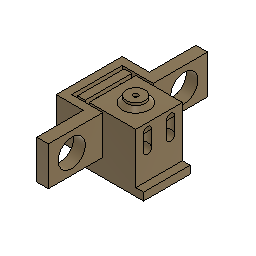
Heatblock+Mk2 (Autodesk Fusion 360 design; units mm, degrees)
Autodesk Fusion 360 part; units mm, degrees
sketch "Sketch1" plane through (0, 0, 0) normal (0, 0, 1) x (1, 0, 0)
  circle A0 centre (0, 0) radius 0.95
  line L0 (-6, 6) -> (6, 6)
  line L1 (6, 6) -> (6, -6)
  line L2 (6, -6) -> (-6, -6)
  line L3 (-6, -6) -> (-6, 6)
  line L4 (-6, 6) -> (6, -6) construction
  line L5 (6, 6) -> (-6, -6) construction
  dimension "d1" = 1.9
  dimension "d2" = 12
  dimension "d3" = 12
  constraint coincident A0.centre origin
  constraint horizontal L0
  constraint perpendicular L0 L1
  constraint parallel L0 L2
  constraint parallel L1 L3
  constraint coincident L4 A0.centre
  constraint coincident L5 A0.centre
  measures "d1" diameter of A0
  measures "d2" distance of L0.end L1.end
  measures "d3" distance of L1.end L2.end
extrude "Extrude1" add sketch "Sketch1" along normal blind 15 makes body 1
ref_plane "WorkPlane1" through (0, 0, 7.5) normal (-1, 0, 0) x (0, -1, 0)
sketch "Sketch2" plane through (0, 1.5, 5) normal (-1, 0, 0) x (0, 1, 0)
  line L0 (-0.55, -10) -> (-2.45, -10)
  line L1 (-7.5, -10) -> (4.5, -10)
  line L2 (4.5, -10) -> (-7.5, -10)
  line L3 (-1.5, -10) -> (-1.5, -12.3) construction
  line L4 (-1.5, -11) -> (-2.1, -11)
  line L5 (-1.5, -11) -> (-0.9, -11)
  line L6 (-0.9, -11) -> (-0.55, -10)
  line L7 (-2.1, -11) -> (-2.45, -10)
  line L8 (-4.9, -10) -> (-3.9, -11)
  line L9 (-3.9, -11) -> (-2.1, -11)
  line L10 (0.9, -11) -> (-0.9, -11)
  line L11 (1.9, -10) -> (0.9, -11)
  line L12 (-0.55, -10) -> (-2.45, -10)
  dimension "d7" = 0.6
  dimension "d23" = 1
  dimension "d24" = 45
  dimension "d25" = 1.8
  constraint midpoint L0 L3.start
  constraint perpendicular L1 L3
  constraint coincident L3 L4.start
  constraint perpendicular L3 L4
  constraint symmetric L3 L4.start L5.start
  constraint symmetric L3 L4.end L5.end
  constraint coincident L0.start L6.end
  constraint coincident L1 L8.start
  constraint parallel L4 L9
  constraint symmetric L3 L8.start L11.start
  constraint symmetric L3 L8.end L10.start
  constraint coincident L0.end L7
  measures "d7" distance of L4.start L4.end
  measures "d23" distance of L1 L9
  measures "d24" angle of L1 L8
  measures "d25" distance of L4.end L8.end
revolve "Revolve1" add sketch "Sketch2" angle 360 about axis through (0, 0, 15) along (0, 0, 1) contours L1 L2 L7 L8 L9 bodies 1
extrude "Extrude2" add 1 faces at (0.149, -1.7888, 16) along direction (0, 0, 1) blind 0.6 on bodies 1 bodies 1
sketch "Sketch3" plane through (6, 0, 0) normal (1, 0, 0) x (0, 1, 0)
  line L0 (-6, 0) -> (6, 0)
  line L1 (6, 15) -> (-6, 15)
  line L2 (-6, 15) -> (-6, 0)
  circle A0 centre (2.95, 13) radius 1.1
  line L3 (-0.95, 0) -> (0.95, 0)
  line L4 (0.95, 15) -> (6, 15)
  line L5 (0.95, 15) -> (0.95, 3) construction
  line L6 (2.95, 13) -> (0.95, 13) construction
  line L7 (2.95, 13) -> (2.95, 15) construction
  line L8 (-0.95, 15) -> (0.95, 15)
  line L9 (6, 0) -> (6, 15)
  line L10 (2.95, 13) -> (2.95, 9) construction
  circle A1 centre (2.95, 9) radius 1.1
  line L11 (0, 15) -> (0, 3.7377) construction
  line L12 (2.95, 9) -> (0.95, 9) construction
  circle A2 centre (-2.95, 13) radius 1.1
  circle A3 centre (-2.95, 9) radius 1.1
  dimension "d11" = 2.2
  dimension "d12" = 2
  dimension "d13" = 2
  dimension "d26" = 2.2
  dimension "d28" = 4
  constraint coincident L1.start L4.end
  constraint perpendicular L4 L5
  constraint coincident A0.centre L6.start
  constraint coincident L5 L6.end
  constraint perpendicular L5 L6
  constraint coincident L1 L7.end
  constraint perpendicular L1 L7
  constraint perpendicular L6 L10
  constraint coincident L10.end A1.centre
  constraint midpoint L8 L11.start
  constraint perpendicular L8 L11
  constraint midpoint L5 L12.end
  constraint horizontal L12
  constraint coincident L4.start L5
  constraint coincident L4.start L5.start
  constraint vertical L5
  constraint symmetric A0 L11 A2
  constraint symmetric A1 L11 A3
  measures "d11" diameter of A0
  measures "d12" distance of A0.centre L7.end
  measures "d13" distance of A0.centre L6.end
  measures "d26" diameter of A1
  measures "d28" distance of A0.centre L10.end
extrude "Extrude3" cut sketch "Sketch3" against normal blind 13.5 contours A0 | A1 | A2 | A3 bodies 1
sketch "Sketch7" plane through (0, -6, 0) normal (0, -1, 0) x (1, 0, 0)
  line L0 (-6, 0) -> (6, 0)
  line L1 (6, 0) -> (6, 15)
  line L2 (6, 15) -> (-6, 15)
  line L3 (-6, 15) -> (-6, 0)
  line L4 (6, 0) -> (8, 0)
  line L5 (8, 0) -> (8, 2)
  line L6 (8, 2) -> (6, 2)
  line L7 (6, 2) -> (6, 0)
  line L8 (-6, 0) -> (-8, 0)
  line L9 (-8, 0) -> (-8, 2)
  line L10 (-8, 2) -> (-6, 2)
  line L11 (-6, 2) -> (-6, 0)
  dimension "d17" = 2
  dimension "d18" = 2
  dimension "d19" = 2
  dimension "d20" = 2
  constraint horizontal L4
  constraint vertical L5
  constraint horizontal L6
  constraint vertical L7
  constraint coincident L0.end L1.start
  constraint horizontal L8
  constraint vertical L9
  constraint horizontal L10
  constraint vertical L11
  constraint coincident L0.start L3.end
  measures "d17" distance of L0.end L4.end
  measures "d18" distance of L0.end L6.end
  measures "d19" distance of L0.start L8.end
  measures "d20" distance of L0.start L10.end
extrude "Extrude4" add sketch "Sketch7" against normal blind 12 contours L3 L8 L9 L10 L11 | L1 L4 L5 L6 L7 bodies 1
sketch "Sketch9" plane through (0, 0, 15) normal (0, 0, 1) x (-1, 0, 0)
  circle A0 centre (0, 0) radius 3.4
  line L0 (6, 6) -> (-6, 6)
  line L1 (-6, 6) -> (-6, -6)
  line L2 (-6, -6) -> (6, -6)
  line L3 (6, -6) -> (6, 6)
  line L4 (-6, 1.85) -> (-6, 4.05)
  line L5 (-6, 6) -> (-6, -6)
  line L6 (-6, -6) -> (-6, 6)
  line L7 (-6, -4.05) -> (-6, -1.85)
  line L8 (-6, 1.85) -> (-6, 4.05)
  line L9 (-6, -4.05) -> (-6, -1.85)
  line L10 (-6, 1.85) -> (-6, 4.05)
  circle A1 centre (-6, 2.95) radius 1.1
  line L11 (-6, 0) -> (-8.5, 0)
  circle A2 centre (-6, -2.95) radius 1.1
  constraint midpoint L4 A1.centre
  constraint coincident L4.start A1
  constraint midpoint L6 L11.start
  constraint perpendicular L6 L11
  constraint symmetric A1 L11 A2
extrude "Extrude5" add sketch "Sketch9" along normal blind -6 and the other way blind 2 separate body contours L1 L4 L5 L6 L8 L10 A1 | L1 L4 L5 L6 L8 L10 A1 | L1 L5 L6 L7 L9 A2 | L1 L5 L6 L7 L9 A2 makes body 2 at (4.9055, -2.8405, 10.3333) makes body 3 at (4.9055, 3.0595, 10.3333)
ref_plane "WorkPlane3" through (0, 0, 7.5) normal (1, 0, 0) x (0, 1, 0)
mirror "Mirror1" about plane through (0, 0, 7.5) normal (1, 0, 0) of bodies 3 2 makes body 4 at (-4.9055, -2.8405, 10.3333) makes body 5 at (-4.9055, 3.0595, 10.3333)
combine "Combine1" operation cut target body 1 tool bodies 4 5 2 3
sketch "Sketch10" plane through (0, 6, 0) normal (0, 1, 0) x (-1, 0, 0)
  line L0 (-8, 0) -> (8, 0)
  line L1 (6, 2) -> (6, 15)
  line L2 (6, 15) -> (-6, 15)
  line L3 (-6, 15) -> (-6, 2)
  line L4 (-6, 15) -> (-7, 15)
  line L5 (-7, 15) -> (-7, 6)
  line L6 (-7, 6) -> (-6, 6)
  line L7 (-6, 6) -> (-6, 15)
  line L8 (-7, 15) -> (-9, 15)
  line L9 (-9, 15) -> (-9, 6)
  line L10 (-9, 6) -> (-7, 6)
  line L11 (-7, 6) -> (-7, 15)
  line L12 (0, 15) -> (0, 11.668)
  line L13 (9, 15) -> (9, 6)
  line L14 (9, 6) -> (7, 6)
  line L15 (7, 6) -> (7, 15)
  line L16 (7, 15) -> (9, 15)
  line L17 (8, 0) -> (8, 2)
  line L18 (8, 2) -> (6, 2)
  line L19 (-6, 2) -> (-8, 2)
  line L20 (-8, 2) -> (-8, 0)
  dimension "d35" = 1
  dimension "d36" = 9
  dimension "d37" = 2
  constraint horizontal L4
  constraint vertical L5
  constraint horizontal L6
  constraint vertical L7
  constraint coincident L2.end L3.start
  constraint horizontal L8
  constraint vertical L9
  constraint horizontal L10
  constraint vertical L11
  constraint midpoint L2 L12.start
  constraint perpendicular L2 L12
  constraint symmetric L4.end L12 L15.end
  constraint symmetric L8.end L12 L13.start
  constraint symmetric L9.end L12 L13.end
  constraint symmetric L5.end L12 L14.end
  measures "d35" distance of L2.end L4.end
  measures "d36" distance of L2.end L6.end
  measures "d37" distance of L4.end L8.end
extrude "Extrude6" add sketch "Sketch10" against normal blind 12 separate body contours L5 L8 L9 L10 L11 makes body 6
sketch "Sketch11" plane through (7, 0, 0) normal (-1, 0, 0) x (0, -1, 0)
  line L0 (-6, 15) -> (-6, 6)
  line L1 (-6, 6) -> (6, 6)
  line L2 (6, 6) -> (6, 15)
  line L3 (6, 15) -> (-6, 15)
  line L4 (-1.85, 13) -> (-1.85, 9)
  arc A0 (-4.05, 9) -> (-1.85, 9) centre (-2.95, 9) ccw
  line L5 (-4.05, 9) -> (-4.05, 13)
  arc A1 (-1.85, 13) -> (-4.05, 13) centre (-2.95, 13) ccw
  line L6 (4.05, 13) -> (4.05, 9)
  arc A2 (1.85, 9) -> (4.05, 9) centre (2.95, 9) ccw
  line L7 (1.85, 9) -> (1.85, 13)
  arc A3 (4.05, 13) -> (1.85, 13) centre (2.95, 13) ccw
  line L8 (-6, 2) -> (6, 2)
  line L9 (6, 2) -> (6, 15)
  line L10 (6, 15) -> (-6, 15)
  line L11 (-6, 15) -> (-6, 2)
  line L12 (-2.95, 13) -> (-2.95, 9) construction
  line L13 (-2.95, 11) -> (2.95, 11) construction
  line L14 (2.95, 13) -> (2.95, 9) construction
  line L15 (-2.95, 10) -> (2.95, 10)
  arc A4 (2.95, 10) -> (2.95, 12) centre (2.95, 11) ccw
  line L16 (2.95, 12) -> (-2.95, 12)
  arc A5 (-2.95, 12) -> (-2.95, 10) centre (-2.95, 11) ccw
  line L17 (-2.95, 11) -> (2.95, 11) construction
  line L18 (-1, 11) -> (-1, 6)
  arc A6 (-1, 6) -> (1, 6) centre (0, 6) ccw
  line L19 (1, 6) -> (1, 11)
  arc A7 (1, 11) -> (-1, 11) centre (0, 11) ccw
  line L20 (0, 11) -> (0, 6) construction
  dimension "d40" = 2
  dimension "d44" = 2
  constraint coincident A1.centre L12.start
  constraint coincident A0.centre L12.end
  constraint midpoint L12 L13.start
  constraint perpendicular L7 L13
  constraint coincident A3.centre L14.start
  constraint coincident A2.centre L14.end
  constraint coincident L13.end L14
  constraint tangent L15 A4
  constraint tangent A4 L16
  constraint parallel L15 L16
  constraint tangent L16 A5
  constraint tangent L15 A5
  constraint coincident L13.end A4.centre
  constraint perpendicular L14 L17
  constraint coincident L13.start A5.centre
  constraint tangent L18 A6
  constraint tangent A6 L19
  constraint parallel L18 L19
  constraint tangent L19 A7
  constraint tangent L18 A7
  constraint perpendicular L15 L20
  constraint midpoint L13 A7.centre
  measures "d40" diameter of A4
  measures "d44" diameter of A6
extrude "Extrude7" cut sketch "Sketch11" against normal blind 1 contours L1 L15 L18 L19 | L15 L18 L19 A7 | L4 L15 L16 L18 A7 | L7 L15 L16 L19 A7 | L4 L15 L16 A5 | L4 A0 L5 A1 L15 L16 A5 | L6 A2 L7 A3 L15 A4 L16 | L7 L15 A4 L16 bodies 6
sketch "Sketch12" plane through (0, 0, 6) normal (0, 0, -1) x (1, 0, 0)
  line L0 (7, 1) -> (8, 1)
  line L1 (8, 1) -> (8, -1)
  line L2 (8, -1) -> (7, -1)
  line L3 (7, -1) -> (7, -6)
  line L4 (7, -6) -> (9, -6)
  line L5 (9, -6) -> (9, 6)
  line L6 (9, 6) -> (7, 6)
  line L7 (7, 6) -> (7, 1)
  line L8 (8, 1) -> (9, 1)
  line L9 (9, 1) -> (9, -1)
  line L10 (9, -1) -> (8, -1)
  line L11 (8, -1) -> (8, 1)
  constraint horizontal L8
  constraint vertical L9
  constraint horizontal L10
  constraint vertical L11
  constraint coincident L5 L9.end
  constraint coincident L0.end L1.start
extrude "Extrude8" cut sketch "Sketch12" against normal blind 1 contours L1 L5 L8 L9 L10 L11 bodies 6
mirror "Mirror2" about plane through (0, 0, 0) normal (1, 0, 0) of bodies 6 makes body 7
move_face "OffsetFaces1" offset -0.3 1 faces at (0, -0.95, 5) on bodies 1
sketch "Sketch13" plane through (0, 0, 15) normal (0, 0, 1) x (-1, 0, 0)
  line L0 (-9, -6) -> (-7, -6)
  line L1 (-7, -6) -> (-7, 6)
  line L2 (-7, 6) -> (-9, 6)
  line L3 (-9, 6) -> (-9, -6)
  circle A0 centre (0, 0) radius 3.4
  line L4 (6, 6) -> (-6, 6)
  line L5 (-6, 6) -> (-6, -6)
  line L6 (-6, -6) -> (6, -6)
  line L7 (6, -6) -> (6, 6)
  line L8 (7, -6) -> (9, -6)
  line L9 (9, -6) -> (9, 6)
  line L10 (9, 6) -> (7, 6)
  line L11 (7, 6) -> (7, -6)
  line L12 (-10, 0.0008) -> (-10, -6.5)
  line L13 (-10, -6.5) -> (0, -6.5)
  line L14 (-11.9999, 0.0008) -> (-11.9999, -8.5001)
  line L15 (-11.9999, -8.5001) -> (-4.9999, -8.5001)
  line L16 (0, -6.5) -> (0, -6)
  line L17 (-11.9999, 0.0008) -> (-13.5981, 0.0008)
  line L18 (-2, -6.5) -> (-5, -6.5)
  line L19 (-4.9999, -8.5001) -> (-5, -8.5001)
  line L20 (-2, -8.4981) -> (-2, -6.5)
  line L21 (-5, -8.5001) -> (-5, -20.4981)
  line L22 (-5, -20.4981) -> (-2, -20.4981)
  line L23 (-2, -20.4981) -> (-2, -8.4981)
  line L24 (-11.9999, 0.0008) -> (-10, 0.0008)
  line L25 (-11.9999, 0.0008) -> (-11.9999, 8.5016)
  line L26 (-4.9999, 8.5016) -> (-5, 8.5016)
  line L27 (-5, 8.5016) -> (-5, 20.4996)
  line L28 (-5, 20.4996) -> (-2, 20.4996)
  line L29 (-2, 20.4996) -> (-2, 8.4996)
  line L30 (-2, 8.4996) -> (-2, 6.5015)
  line L31 (-11.9999, 8.5016) -> (-4.9999, 8.5016)
  line L32 (-11.9999, 0.0008) -> (-10, 0.0008)
  line L33 (-10, 0.0008) -> (-10, 6.5015)
  line L34 (-10, 6.5015) -> (0, 6.5015)
  line L35 (0, 6.5015) -> (-2.0442, 6.5014)
  line L36 (-5, 8.5016) -> (-4.9999, 6.5013)
  line L37 (-5, 8.5016) -> (-2, 8.4996)
  line L38 (-2, 6.5015) -> (-2.1288, 6.5012)
  line L39 (0, -6.5) -> (-5, -6.5)
  dimension "d52" = 2
  dimension "d53" = 3
  dimension "d54" = 12
  dimension "d60" = 0.5
  dimension "d61" = 7
  dimension "d62" = 6.5008
  dimension "d63" = 8.5009
  dimension "d64" = 1.9999
  constraint midpoint L6 L16.end
  constraint perpendicular L6 L16
  constraint parallel L3 L14
  constraint parallel L0 L15
  constraint perpendicular L12 L17
  constraint parallel L3 L12
  constraint parallel L0 L13
  constraint horizontal L18
  constraint horizontal L19
  constraint vertical L20
  constraint vertical L21
  constraint horizontal L22
  constraint vertical L23
  constraint perpendicular L12 L24
  constraint symmetric L13.end L17 L34.end
  constraint symmetric L12.end L17 L33.end
  constraint symmetric L15.end L17 L26.start
  constraint symmetric L14.end L17 L25.end
  constraint symmetric L12.start L17 L24.end
  constraint symmetric L17 L14.start L24.start
  constraint symmetric L17 L18.start L30.end
  constraint symmetric L17 L20.start L29.end
  constraint symmetric L17 L19.end L26.end
  constraint symmetric L17 L21.end L27.end
  constraint symmetric L17 L22.end L28.end
  constraint coincident L35 L36.end
  constraint perpendicular L35 L36
  constraint coincident L38 L35.end
  constraint horizontal L39
  constraint coincident L13.end L16.start
  measures "d52" distance of L13.end L18.start
  measures "d53" distance of L20.start L19.end
  measures "d54" distance of L20.start L22.end
  measures "d60" distance of L13.end L16.end
  measures "d61" distance of L15.end L14.end
  measures "d62" distance of L12.end L12.start
  measures "d63" distance of L14.end L14.start
  measures "d64" distance of L12 L14
extrude "Extrude9" add sketch "Sketch13" against normal blind 10 separate body contours L12 L13 L14 L15 L18 L20 L21 L22 L23 L24 L32 L39 | L24 L25 L31 L32 L33 L34 L36 | L30 L34 L35 L36 L37 L38 | L27 L28 L29 L37 makes body 8
sketch "Sketch14" plane through (5, 0, 0) normal (1, 0, 0) x (0, 1, 0)
  line L0 (-8.5016, 15) -> (-20.4996, 15)
  line L1 (-20.4996, 15) -> (-20.4996, 5)
  line L2 (-20.4996, 5) -> (-8.5016, 5)
  line L3 (-8.5016, 5) -> (-8.5016, 15)
  line L4 (-20.4996, 15) -> (-8.5016, 5) construction
  circle A0 centre (-14.5006, 10) radius 3.5
  line L5 (8.5001, 15) -> (-8.5016, 15)
  line L6 (-8.5016, 15) -> (-8.5016, 5)
  line L7 (-8.5016, 5) -> (8.5001, 5)
  line L8 (8.5001, 5) -> (8.5001, 15)
  line L9 (-0.0008, 5) -> (-0.0008, 9.1854)
  circle A1 centre (14.4991, 10) radius 3.5
  line L10 (20.4981, 15) -> (8.5001, 5) construction
  dimension "d57" = 7
  constraint coincident L0.end L1.start
  constraint coincident L2.end L3.start
  constraint midpoint L4 A0.centre
  constraint midpoint L7 L9.start
  constraint perpendicular L7 L9
  constraint symmetric L0.end L9 L10.start
  constraint symmetric L2.end L9 L7.end
  constraint symmetric A0 L9 A1
  measures "d57" diameter of A0
extrude "Extrude10" cut sketch "Sketch14" against normal blind 4 contours A0 | A1 bodies 8
mirror "Mirror3" about plane through (0, 0, 7.5) normal (1, 0, 0) of bodies 8 makes body 9
hidden bodies 6 8
named bodies: "Hotend Mk2", "Connection Clamp Right", "Connection Clamp Left", "Clamp", "Clamp (1)"
